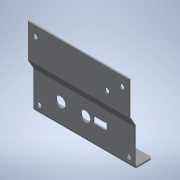
# Autodesk Inventor part: Enclosure-Cap
Saved by Autodesk Inventor 2022 (Build 260153000, 153)
## iProperties
Created: 2024-04-02
Part Number: Enclosure-Cap
Material: Generic
Document SubType Name: Sheet Metal
Designer: Baaij
Density: 1 g/cm^3
Sheet Metal Rule: Default_mm
Appearance: Default
Flat Pattern Width: 6.85312 cm
Flat Pattern Length: 7.1 cm
Flat Pattern Area: 48.6572 cm^2
Sheet Metal Width: 68.531 mm
Sheet Metal Length: 71.000 mm
Sheet Metal Area: 4865.716 mm^2
Author: Baaij
Autodesk Inventor part; units mm, degrees
ref_plane "YZ Plane" through (0, 0, 0) normal (1, 0, 0) x (0, 1, 0)
ref_plane "XZ Plane" through (0, 0, 0) normal (0, 1, 0) x (-1, 0, 0)
ref_plane "XY Plane" through (0, 0, 0) normal (0, 0, 1) x (1, 0, 0)
sketch "Sketch1" plane through (0, 0, 0) normal (0, 0, 1) x (1, 0, 0)
  line L0 (0, 18.2) -> (0, -18.2) construction
  line L1 (-49.7, 0) -> (49.7, 0) construction
  line L2 (-35.5, 13) -> (35.5, 13)
  line L3 (35.5, 13) -> (35.5, -13)
  line L4 (35.5, -13) -> (-35.5, -13)
  line L5 (-35.5, -13) -> (-35.5, 13)
  line L6 (-35.5, 13) -> (35.5, -13) construction
  line L7 (35.5, 13) -> (-35.5, -13) construction
  line L8 (14.985, 5.1105) -> (14.985, 5.5105) projected
  line L9 (14.985, 5.1105) -> (7.455, 5.1105) projected
  line L10 (7.455, 5.5105) -> (7.455, 5.1105) projected
  line L11 (6.455, 5.5105) -> (7.455, 5.5105) projected
  line L12 (6.455, 0.7105) -> (6.455, 5.5105) projected
  line L13 (6.455, 0.7105) -> (15.985, 0.7105) projected
  line L14 (15.985, 0.7105) -> (15.985, 5.5105) projected
  line L15 (14.985, 5.5105) -> (15.985, 5.5105) projected
  point P0 (0, 0)
  dimension "d0" = 71
  dimension "d1" = 26
  constraints: 12 end point, 2 midpoint, 2 parallel, 1 horizontal, 1 perpendicular
  measures "d0" distance of L3.end L4.end
  measures "d1" distance of L2.end L3.end
extrude "Plate1" add sketch "Sketch1" along normal blind 1
sketch "Sketch2" plane through (-35.5, 13.5, 1.134) normal (0, 0.5, -0.8660254) x (-1, 0, 0)
  line L0 (-71, 0) -> (0, 0)
  line L1 (0, 0) -> (0, 7.4641)
  line L2 (0, 7.4641) -> (-71, 7.4641)
  line L3 (-71, 7.4641) -> (-71, 0)
  constraints: 6 end point, 1 horizontal, 1 perpendicular, 1 vertical
edge flange "Flange1" height 8 angle 30 thickness 1 bend radius 1 thickness toward (0, 0.5, -0.8660254) relief tear relief width 1 relief depth 0.5 edges at (0, 13, 1) wall of the first edge with corners at (35.5, 13.5, 1.134) (-35.5, 13.5, 1.134) (-35.5, 19.9641, 4.866) (35.5, 19.9641, 4.866)
bend "Bend1"
corner "Corner1"
sketch "Sketch3" plane through (35.5, 19.9641, 3.866) normal (0, 0, 1) x (1, 0, 0)
  line L0 (-71, 0) -> (0, 0)
  line L1 (0, 0) -> (0, 23.869)
  line L2 (0, 23.869) -> (-71, 23.869)
  line L3 (-71, 23.869) -> (-71, 0)
  constraints: 6 end point, 1 horizontal, 1 perpendicular, 1 vertical
edge flange "Flange2" height 23.869 angle 30 thickness 1 bend radius 1 thickness toward (0, 0, 1) relief tear relief width 1 relief depth 0.5 edges at (0, 20.4641, 4) wall of the first edge with corners at (-35.5, 19.9641, 3.866) (35.5, 19.9641, 3.866) (35.5, 43.8331, 3.866) (-35.5, 43.8331, 3.866)
bend "Bend2"
corner "Corner2"
sketch "Sketch4" plane through (-35.5, -12, 1) normal (0, -1, 0) x (1, 0, 0)
  line L0 (71, 0) -> (0, 0)
  line L1 (0, 0) -> (0, -12.5)
  line L2 (0, -12.5) -> (71, -12.5)
  line L3 (71, -12.5) -> (71, 0)
  constraints: 6 end point, 1 horizontal, 1 perpendicular, 1 vertical
edge flange "Flange3" height 12.5 angle 90 thickness 1 bend radius 1 thickness toward (0, -1, 0) relief tear relief width 1 relief depth 0.5 edges at (0, -13, 0) wall of the first edge with corners at (35.5, -12, 1) (-35.5, -12, 1) (-35.5, -12, -11.5) (35.5, -12, -11.5)
bend "Bend3"
corner "Corner3"
fillet "Fillet1" radius 1.5 2 edges at (-35.5, -12.5, -11.5) (35.5, -12.5, -11.5)
sketch "Sketch5" plane through (-35.5, 43.8331, 4.866) normal (0, 0, 1) x (1, 0, 0)
  circle A0 centre (5, -7.1331) radius 1.6 projected
  circle A1 centre (66, -7.1331) radius 1.6 projected
  circle A2 centre (55.5, -14.8331) radius 1.5 projected
  point P0 (35.5, -43.8331)
hole "Hole3" at (-30.5, 36.7, 4.866) at (20, 29, 4.866) at (30.5, 36.7, 4.866) direction (0, 0, -1) diameter 3.2 end through all
sketch "Sketch6" plane through (0, 0, 1) normal (0, 0, 1) x (1, 0, 0)
  circle A0 centre (-16.48, 2) radius 2.286 projected
  circle A1 centre (1.02, 2) radius 2.286 projected
  circle A2 centre (-31.5, -7.5) radius 1.6 projected
  circle A3 centre (31.5, -7.5) radius 1.6 projected
  point P0 (0, 0)
hole "Hole4" at (-31.5, -7.5, 1) at (31.5, -7.5, 1) direction (0, 0, -1) diameter 3.2 end through all
hole "Hole5" at (1.02, 2, 1) at (-16.48, 2, 1) direction (0, 0, -1) diameter 7 end through all
equation "\"d62\" = Thickness"
equation "\"d2\" = Thickness"
equation "\"d3\" = BendReliefWidth"
equation "\"d4\" = BendReliefDepth"
equation "\"d5\" = MinimumRemnant"
equation "\"d6\" = TransitionRadius"
equation "\"d9\" = BendRadius"
equation "\"d10\" = CornerReliefSize"
equation "\"d11\" = GapSize"
equation "\"d12\" = JacobiRadiusSize"
equation "\"d13\" = BendReliefWidth"
equation "\"d14\" = BendReliefDepth"
equation "\"d15\" = MinimumRemnant"
equation "\"d16\" = TransitionRadius"
equation "\"d19\" = BendRadius"
equation "\"d20\" = CornerReliefSize"
equation "\"d21\" = GapSize"
equation "\"d22\" = JacobiRadiusSize"
equation "\"d23\" = BendReliefWidth"
equation "\"d24\" = BendReliefDepth"
equation "\"d25\" = MinimumRemnant"
equation "\"d26\" = TransitionRadius"
equation "\"d29\" = BendRadius"
equation "\"d30\" = CornerReliefSize"
equation "\"d31\" = GapSize"
equation "\"d32\" = JacobiRadiusSize"
equation "\"BendRadius\" = Thickness"
equation "\"BendReliefWidth\" = Thickness"
equation "\"BendReliefDepth\" = 0.5 * Thickness"
equation "\"CornerReliefSize\" = 4 * Thickness"
equation "\"MinimumRemnant\" = 2 * Thickness"
equation "\"TransitionRadius\" = BendRadius"
equation "\"JacobiRadiusSize\" = BendRadius"
equation "\"GapSize\" = Thickness"
equation "\"Thickness\" = 1"
body "Solid1"
